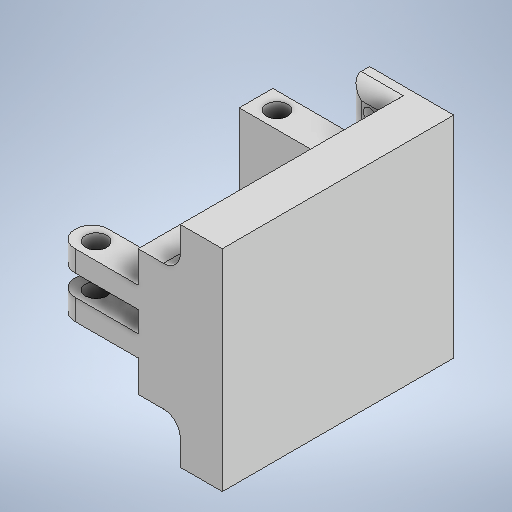
# Autodesk Inventor part: SuspensionSupporter
Saved by Autodesk Inventor 2025.2 (Build 292293000, 293)
## iProperties
Created: 2025-01-03
Part Number: SuspensionSupporter
Material: 일반
Document SubType Name: Modeling
Designer: SEON
Density: 1 g/cm^3
Appearance: 기본값
Author: SEON
Autodesk Inventor part; units mm, degrees
ref_plane "YZ Plane" through (0, 0, 0) normal (1, 0, 0) x (0, 1, 0)
ref_plane "XZ Plane" through (0, 0, 0) normal (0, 1, 0) x (-1, 0, 0)
sketch "스케치1" plane through (0, 0, 0) normal (0, 0, 1) x (1, 0, 0)
  line L0 (-20, -25) -> (20, -25)
  line L1 (20, -25) -> (20, 25)
  line L2 (20, 25) -> (-20, 25)
  line L3 (-20, 25) -> (-20, -25)
  line L4 (-20, -25) -> (20, 25) construction
  line L5 (20, -25) -> (-20, 25) construction
  circle A0 centre (-15, 20) radius 1.5
  circle A1 centre (-15, -20) radius 1.5
  circle A2 centre (15, 20) radius 1.5
  circle A3 centre (15, -20) radius 1.5
  line L6 (0, 25) -> (0, -25)
  point P0 (0, 0)
  point P1 (-20, 0)
  dimension "d0" = 40
  dimension "d1" = 50
  dimension "d2" = 30
  dimension "d3" = 15
  dimension "d4" = 40
  dimension "d6" = 20
  dimension "d7" = 3
  constraints: 14 end point, 5 midpoint, 4 centre point, 3 equal radius, 2 horizontal alignment, 2 parallel, 2 vertical alignment, 1 horizontal, 1 perpendicular
  measures "d0" distance of L1.end L2.end
  measures "d1" distance of L2.end L0.start
  measures "d2" distance of A2.centre A0.centre
  measures "d3" horizontal distance of L6.start A0.centre
  measures "d4" distance of A1.centre A0.centre
  measures "d6" vertical distance of point (-20, 0) A0.centre
  measures "d7" diameter of A0
extrude "돌출1" add sketch "스케치1" along normal blind 5 contours L3 L2 L6 L0
sketch "스케치2" plane through (0, 0, 5) normal (0, 0, 1) x (1, 0, 0)
  circle A0 centre (15, -20) radius 1.5 projected
  circle A1 centre (-15, -20) radius 1.5 projected
  line L0 (0, 25) -> (-20, 25) projected
  line L1 (-20, 25) -> (-20, -25) projected
  line L2 (-20, -25) -> (0, -25) projected
  circle A2 centre (-15, 20) radius 1.5 projected
  circle A3 centre (-15, -20) radius 1.5 projected
  line L3 (-20, -25) -> (20, -25) projected
  line L4 (14, -15) -> (20, -15)
  line L5 (10, -25) -> (10, -19)
  arc A4 (14, -15) -> (10, -19) centre (14, -19) ccw
  line L6 (-28, 0) -> (28, 0) projected
  line L7 (0, -35) -> (0, 35) projected
  line L8 (-14, -15) -> (-20, -15)
  line L9 (-10, -25) -> (-10, -19)
  arc A5 (-10, -19) -> (-14, -15) centre (-14, -19) ccw
  line L10 (14, 15) -> (20, 15)
  line L11 (10, 25) -> (10, 19)
  arc A6 (10, 19) -> (14, 15) centre (14, 19) ccw
  line L12 (-10, 25) -> (-10, 19)
  arc A7 (-14, 15) -> (-10, 19) centre (-14, 19) ccw
  line L13 (-14, 15) -> (-20, 15)
  line L14 (0, -25) -> (0, 25) projected
  point P0 (10, -15)
  point P1 (0, 0)
  dimension "d13" = 10
  dimension "d16" = 4
  constraints: 16 end point, 15 symmetric about line, 8 point on circle, 4 centre point, 3 point on line, 2 tangent, 1 vertical, 3 other
  measures "d13" distance between parallel lines of L2 L4
  measures "d16" radius of A4
extrude "돌출2" add sketch "스케치2" along normal blind 50 contours L7 L6 L1 L13 A7 L12 L0 | L7 L2 L9 A5 L8 L1 L6
fillet "모깎기1" radius 3 4 edges at (-15, -25, 5) (-20, -20, 5) (-15, 25, 5) (-20, 20, 5)
sketch "스케치3" plane through (-20, -25, 0) normal (-1, 0, 0) x (0, 0, 1)
  line L0 (2, 40) -> (55, 40) projected
  line L1 (5, 10) -> (55, 10) projected
  line L2 (4, 40) -> (12, 40)
  line L3 (12, 40) -> (12, 10)
  line L4 (12, 10) -> (4, 10)
  line L5 (4, 10) -> (4, 40)
  line L6 (0, 50) -> (0, 0) projected
  line L7 (12, 32) -> (4, 32)
  line L8 (4, 32) -> (4, 18)
  line L9 (4, 18) -> (12, 18)
  line L10 (12, 18) -> (12, 32)
  line L11 (12, 38) -> (4, 38)
  line L12 (4, 38) -> (4, 12)
  line L13 (4, 12) -> (12, 12)
  line L14 (12, 12) -> (12, 38)
  point P0 (0, 25)
  point P1 (15, 10)
  point P2 (12, 25)
  point P3 (4, 25)
  point P4 (12, 18)
  point P5 (12, 25)
  point P6 (8, 12)
  dimension "d17" = 8
  dimension "d18" = 4
  dimension "d21" = 8
  dimension "d28" = 26
  constraints: 24 end point, 6 parallel, 6 point on line, 5 midpoint, 3 horizontal, 3 perpendicular, 1 horizontal alignment
  measures "d17" distance between parallel lines of L5 L3
  measures "d18" distance between parallel lines of L6 L5
  measures "d21" distance between parallel lines of L0 L7
  measures "d28" distance from line of point (8, 12) L11
extrude "돌출3" add sketch "스케치3" along normal blind 19 contours L11 L3 L7 L5 | L7 L3 L9 L5 | L9 L3 L13 L5
sketch "스케치5" plane through (-20, -13, 4) normal (0, -1, 0) x (1, 0, 0)
  circle A0 centre (-14, 4) radius 2.5
  line L0 (-19, 0) -> (-19, 8) projected
  point P0 (20, -4)
  point P1 (-19, 4)
  dimension "d29" = 5
  dimension "d30" = 5
  constraints: 1 centre point, 1 horizontal alignment, 1 midpoint
  measures "d29" diameter of A0
  measures "d30" distance from line of L0 A0.centre
extrude "돌출5" cut sketch "스케치5" against normal through all
ref_plane "작업 평면1" through (-20, 0, 0) normal (0, -1, 0) x (1, 0, 0)
sketch "스케치6" plane through (-20, 0, 0) normal (0, -1, 0) x (1, 0, 0)
  line L0 (0, 2) -> (0, 55) projected
  line L1 (0, 55) -> (-19, 55)
  line L2 (-19, 55) -> (-19, 47)
  line L3 (-19, 47) -> (0, 47)
  line L4 (0, 47) -> (0, 55)
  line L5 (-19, 12) -> (-19, 4) projected
  circle A0 centre (-14, 51) radius 2.5
  circle A1 centre (-14, 8) radius 2.5 projected
  point P0 (20, 0)
  point P1 (0, 47)
  dimension "d31" = 0
  dimension "d33" = 8
  dimension "d34" = 8
  dimension "d35" = 4
  constraints: 8 end point, 2 parallel, 2 vertical alignment, 1 centre point, 1 equal radius, 1 horizontal, 1 perpendicular
  measures "d33" distance of L5.start L5.end
  measures "d34" distance of L1.end L2.end
  measures "d35" distance from line of A0.centre L1
extrude "돌출6" add sketch "스케치6" along normal mid plane 15 contours L3 L2 L1 L0
extrude "돌출7" cut sketch "스케치6" along normal mid plane 5 contours L3 L2 L1 L0
fillet "모깎기2" radius 4 4 edges at (-39, 5, 55) (-39, 5, 47) (-39, -5, 55) (-39, -5, 47)
equation "\"d3\" = 0.5 * d2"
equation "\"d6\" = 0.5 * d4"
equation "\"d34\" = d33"
equation "\"d35\" = 0.5 * d34"
